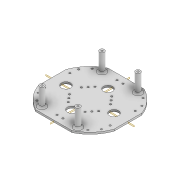
# Autodesk Inventor part: Drone_plate_2
Saved by Autodesk Inventor 2022 (Build 260153000, 153)
## iProperties
Created: 2022-04-28
Part Number: Drone_plate_2
Material: Generic
Document SubType Name: Modeling
Designer: dell
Density: 1 g/cm^3
Appearance: Default
Mass: 78.55 g
Surface Area: 799.842 cm^2
Volume: 78.55 cm^3
Author: dell
Autodesk Inventor part; units mm, degrees
ref_plane "XZ Plane" through (0, 0, 0) normal (0, 1, 0) x (-1, 0, 0)
ref_plane "XY Plane" through (0, 0, 0) normal (0, 0, 1) x (1, 0, 0)
sketch "Sketch1" plane through (0, 0, 0) normal (0, 1, 0) x (-1, 0, 0)
  line L0 (0, 0) -> (60, 0)
  line L1 (60, 0) -> (60, -120)
  line L2 (60, -120) -> (0, -120)
  line L3 (0, -120) -> (0, 0)
  line L4 (60, 0) -> (0, -120) construction
  line L5 (60, -120) -> (0, 0) construction
  circle A0 centre (30, -60) radius 67.082
  line L6 (30, -120) -> (30, 7.082) construction
  line L7 (60, -60) -> (0, -60)
  line L8 (30, -60) -> (81.3878, -103.1195) construction
  circle A1 centre (82.6371, -93.7245) radius 1.5
  circle A2 centre (54.2934, -69.9413) radius 1.5
  line L9 (41.76, -45.985) -> (17.4815, -74.919) construction
  circle A3 centre (72.3525, -105.9812) radius 1.5
  circle A4 centre (44.0088, -82.198) radius 1.5
  line L10 (-33, -36.9566) -> (-33, -83.0434)
  line L11 (93, -36.9566) -> (93, -83.0434)
  circle A5 centre (49.1511, -76.0697) radius 1.5
  circle A6 centre (60, -110) radius 1.5
  circle A7 centre (70, -60) radius 7.5
  circle A8 centre (30, -90) radius 7.5
  circle A9 centre (84.4498, -80.8618) radius 1.5
  point P0 (60, -120)
  point P1 (60, 0)
  point P2 (30, -60)
  dimension "d0" = 120
  dimension "d25" = 60
  dimension "d27" = 50
  dimension "d28" = 3
  dimension "d30" = 3
  dimension "d32" = 25
  dimension "d33" = 62
  dimension "d34" = 8
  dimension "d35" = 8
  dimension "d38" = 63
  dimension "d39" = 63
  dimension "d40" = 3
  dimension "d41" = 25
  dimension "d50" = 3
  dimension "d51" = 10
  dimension "d52" = 15
  dimension "d53" = 40
  dimension "d54" = 15
  dimension "d55" = 30
  constraints: 24 end point, 9 centre point, 6 midpoint, 4 point on line, 3 parallel, 3 perpendicular, 3 symmetric about line, 1 coincident, 1 horizontal, 1 horizontal alignment, 1 vertical, 12 other
  measures "d0" distance of L2.end L0.start
  measures "d25" distance between parallel lines of L1 L3
  measures "d27" angle of L6 L8
  measures "d28" diameter of A1
  measures "d30" diameter of A2
  measures "d32" distance from line of L9 A2.centre
  measures "d33" distance from line of L9 A1.centre
  measures "d34" distance from line of L8 A2.centre
  measures "d35" distance from line of L8 A1.centre
  measures "d38" distance from line of point (30, -60) L10
  measures "d39" distance from line of point (30, -60) L11
  measures "d40" diameter of A5
  measures "d41" distance of L8.start A5.centre
  measures "d50" diameter of A6
  measures "d51" distance of L1.end A6.centre
  measures "d52" diameter of A7
  measures "d53" distance of L8.start A7.centre
  measures "d54" diameter of A8
  measures "d55" distance of L8.start A8.centre
extrude "Extrusion1" add sketch "Sketch1" along normal blind 3 contours L0 L1 L7 L3 | L3 A0 L10 | A0 L11 L1 A6 | L7 L1 A6 L2 L3 | A6 L1 | L1 A6 | A1 | A2 | A3 | A4 | A5 | A7 | A8 | A9
extrude "Extrusion3" cut sketch "Sketch1" along normal blind 10 contours A6 L1 | L1 A6 | A1 | A2 | A3 | A4 | A5 | A7 | A8 | A9
ref_plane "Work Plane5" through (-60, 0, -60) normal (0, 0, 1) x (1, 0, 0)
ref_plane "Work Plane6" through (-30, 0, 0) normal (1, 0, 0) x (0, 1, 0)
mirror "Mirror3" about plane through (-60, 0, -60) normal (0, 0, 1) of "Extrusion3"
mirror "Mirror4" about plane through (-30, 0, 0) normal (1, 0, 0) of "Extrusion3", "Mirror3"
sketch "Sketch7" plane through (0, 0, 0) normal (0, -1, 0) x (1, 0, 0)
  circle A0 centre (-25.05, -110) radius 1.5
  circle A1 centre (-34.95, -110) radius 1.5
  line L0 (0, -120) -> (-60, -120) projected
  line L1 (-30, 28.4216) -> (-30, -148.4216) projected
  point P0 (0, 0)
  dimension "d42" = 3
  dimension "d43" = 3
  dimension "d44" = 10
  dimension "d45" = 10
  dimension "d46" = 4.95
  dimension "d47" = 4.95
  constraints: 2 centre point
  measures "d42" diameter of A0
  measures "d43" diameter of A1
  measures "d44" distance from line of L0 A0.centre
  measures "d45" distance from line of L0 A1.centre
  measures "d46" distance from line of L1 A0.centre
  measures "d47" distance from line of L1 A1.centre
extrude "Extrusion4" cut sketch "Sketch7" against normal blind 100
mirror "Mirror5" about plane through (-60, 0, -60) normal (0, 0, 1) of "Extrusion4"
sketch "Sketch9" plane through (0, 3, 0) normal (0, 1, 0) x (1, 0, 0)
  circle A0 centre (-34.95, 10) radius 1.5 projected
  circle A1 centre (-25.05, 10) radius 1.5 projected
  circle A2 centre (-34.95, 110) radius 1.5 projected
  circle A3 centre (-25.05, 110) radius 1.5 projected
  circle A4 centre (22.6371, 26.2755) radius 1.5 projected
  circle A5 centre (-15.9912, 37.802) radius 1.5 projected
  circle A6 centre (0, 10) radius 1.5 projected
  circle A7 centre (12.3525, 14.0188) radius 1.5 projected
  circle A8 centre (-5.7066, 50.0587) radius 1.5 projected
  circle A9 centre (-10.8489, 43.9303) radius 1.5 projected
  circle A10 centre (24.4498, 39.1382) radius 1.5 projected
  circle A11 centre (22.6371, 93.7245) radius 1.5 projected
  circle A12 centre (-15.9912, 82.198) radius 1.5 projected
  circle A13 centre (0, 110) radius 1.5 projected
  circle A14 centre (10, 60) radius 7.5 projected
  circle A15 centre (12.3525, 105.9812) radius 1.5 projected
  circle A16 centre (-5.7066, 69.9413) radius 1.5 projected
  circle A17 centre (-10.8489, 76.0697) radius 1.5 projected
  circle A18 centre (24.4498, 80.8618) radius 1.5 projected
  circle A19 centre (-30, 30) radius 7.5 projected
  circle A20 centre (-82.6371, 26.2755) radius 1.5 projected
  circle A21 centre (-44.0088, 37.802) radius 1.5 projected
  circle A22 centre (-60, 10) radius 1.5 projected
  circle A23 centre (-72.3525, 14.0188) radius 1.5 projected
  circle A24 centre (-54.2934, 50.0587) radius 1.5 projected
  circle A25 centre (-49.1511, 43.9303) radius 1.5 projected
  circle A26 centre (-84.4498, 39.1382) radius 1.5 projected
  circle A27 centre (-30, 90) radius 7.5 projected
  circle A28 centre (-82.6371, 93.7245) radius 1.5 projected
  circle A29 centre (-44.0088, 82.198) radius 1.5 projected
  circle A30 centre (-60, 110) radius 1.5 projected
  circle A31 centre (-70, 60) radius 7.5 projected
  circle A32 centre (-72.3525, 105.9812) radius 1.5 projected
  circle A33 centre (-54.2934, 69.9413) radius 1.5 projected
  circle A34 centre (-49.1511, 76.0697) radius 1.5 projected
  circle A35 centre (-84.4498, 80.8618) radius 1.5 projected
  line L0 (0, 120) -> (-60, 120) projected
  arc A36 (-60, 120) -> (-93, 83.0434) centre (-30, 60) ccw projected
  line L1 (-93, 83.0434) -> (-93, 36.9566) projected
  arc A37 (-93, 36.9566) -> (-60, 0) centre (-30, 60) ccw projected
  line L2 (-60, 0) -> (0, 0) projected
  arc A38 (0, 0) -> (33, 36.9566) centre (-30, 60) ccw projected
  line L3 (33, 36.9566) -> (33, 83.0434) projected
  arc A39 (33, 83.0434) -> (0, 120) centre (-30, 60) ccw projected
  circle A40 centre (-60, 10) radius 1.5 projected
  circle A41 centre (-60, 10) radius 4
  circle A42 centre (-60, 110) radius 1.5 projected
  circle A43 centre (-60, 110) radius 4
  circle A44 centre (0, 110) radius 1.5 projected
  circle A45 centre (0, 110) radius 4
  circle A46 centre (0, 10) radius 4
  circle A47 centre (0, 10) radius 1.6
  circle A48 centre (0, 110) radius 1.6
  circle A49 centre (-60, 110) radius 1.6
  circle A50 centre (-60, 10) radius 1.6
  dimension "d56" = 8
  dimension "d57" = 8
  dimension "d58" = 8
  dimension "d59" = 8
  dimension "d60" = 0.1
  dimension "d61" = 0.1
  dimension "d62" = 0.1
  dimension "d63" = 0.1
  constraints: 8 centre point, 4 coincident
  measures "d56" diameter of A41
  measures "d57" diameter of A43
  measures "d58" diameter of A45
  measures "d59" diameter of A46
  measures "d60" radial gap between concentric circles of A6 A47
  measures "d61" radial gap between concentric circles of A13 A48
  measures "d62" radial gap between concentric circles of A30 A49
  measures "d63" radial gap between concentric circles of A22 A50
extrude "Extrusion5" cut sketch "Sketch9" against normal blind 10 contours A47 | A48 | A49 | A50
extrude "Extrusion6" add sketch "Sketch9" along normal blind 30 contours A41 | A43 | A45 | A46
fillet "Fillet2" radius 3 4 edges at (-4, 3, -10) (-64, 3, -10) (-4, 3, -110) (-64, 3, -110)
equation "\"d45\" = d44"
equation "\"d47\" = d46"
body "Solid1"
